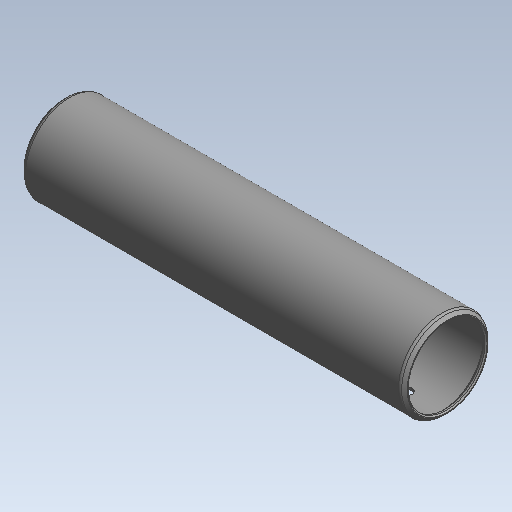
# Autodesk Inventor part: 04-3.4462C
Saved by Autodesk Inventor 2020 (Build 240168000, 168)
## iProperties
Part Number: 04-3.4462C
Material: Generic
Catalog Web Link: www.cadenas.de
Description: Tube-Original Line - Standard Air Cylinders
Vendor: BIMBA
Document SubType Name: Modeling
Designer: partserver
Manufacturer: BIMBA
Mass: 3.10241 g
Surface Area: 111.945 cm^2
Volume: 3.10241 cm^3
Density: 1 g/cm^3
Appearance: PSOLRGB-180-180-180
Category: PARTsolutions
Company: BIMBA
PSOL_IDENT_0: {$CADENAS_DATA\23d-libs\bimba\bimba_brand\bimba_imperial\bimba_full_line\original_line_cylinders\sta
PSOL_IDENT_1: ndard_air_cylinders\tube.prj},199 {VTYP=3D},{NB=04-3.4462C},{LINA=04-3.4462C},{NN=Tube},{DATE=19.01.
PSOL_IDENT_2: 2022 10:19:38},{GEOMDATE=03.03.2020 12:52:40},{VERSION=},{LINEID=40},{WBVAR=MNT,ACTING,NR,L,FOURHOLE
PSOL_IDENT_3: S,SR,K},{WBNUMERIC=L,FOURHOLES}  {NB=04-3.4462C},{LINA=04-3.4462C},{KT=DUMMY},{PN=04-3.4462C},{BORE=
PSOL_IDENT_4: 0.75000000},{BOREPN=04},{MNT=},{MNTALG='' , 'Front Nose' , 'BF' , 'Front Block' , 'BFT' , 'Front Tru
PSOL_IDENT_5: nnion' , 'A' , 'Adjustable Stroke'},{ACTING=},{ACTINGALG= '' , 'Single Acting' , 'R' , 'Reverse/Doub
PSOL_IDENT_6: le Acting' },{NR=},{NRALG= '' , 'Without Non-rotating Rod' , 'NR' , 'With Non-rotating Rod' },{L=3.4
PSOL_IDENT_7: 460},{OD=0.8050},{ODN=0.8050},{ODP=0.8625},{ODB=0.8325},{ID=0.7615},{DV=0.00000000},{LV=0.00000000},
PSOL_IDENT_8: {LV1=0.00000000},{G=0.0300},{FOURHOLES=2},{AA=0.3750},{BB=0.0940},{SR=C},{SRALG= 'C' , 'Carbon Steel
PSOL_IDENT_9: Rod' , 'SR' , '303 Stainless Steel Rod' , '' , '303 Stainless Steel Rod'},{KALG= '', 'Standard' , '
PSOL_IDENT_10: K' , 'Ports Rotated 90deg' },{K=}
NB: 04-3.4462C
NN: Tube
NT: Original Line - Standard Air Cylinders
NBSYN: $PN.
LINA: 04-3.4462C
CATALOG: Bimba Products
BORE: 0
BOREPN: 04
MNT: Front Nose
MNTALG: '' , 'Front Nose' , 'BF' , 'Front Block' , 'BFT' , 'Front Trunnion' , 'A' , 'Adjustable Stroke'
ACTING: Single Acting
NR: Without Non-rotating Rod
L: 3.446
ODN: 0.805
ODP: 0.8625
ODB: 0.8325
ID: 0.7615
DV: 0
LV: 0
LV1: 0
G: 0.03
FOURHOLES: 2
AA: 0.375
BB: 0.094
SR: Carbon Steel Rod
K: Standard
SUPPLIER: BIMBA
ARTICLENO: 04-3.4462C
BOMINFO: 04-3.4462C
CREATOR: CADENAS GmbH
Title: 04-3.4462C
Author: Cadenas PARTsolutions
Comments: Original Line - Standard Air Cylinders
Autodesk Inventor part; units mm, degrees
sketch "Sketch_1" plane through (0, 0, 0) normal (0, 0, 1) x (1, 0, 0)
  line L0 (87.5284, 0) -> (0, 0)
  arc A0 (-0.6395, 9.3472) -> (-0.6395, 9.1676) centre (-0.5497, 9.2574) ccw
  line L1 (-0.6395, 9.1676) -> (-0.381, 8.9091)
  line L2 (-0.381, 8.9091) -> (0, 8.9091)
  line L3 (0, 8.9091) -> (0.762, 9.671)
  line L4 (0.762, 9.671) -> (86.7664, 9.671)
  line L5 (86.7664, 9.671) -> (87.5284, 8.9091)
  line L6 (87.5284, 8.9091) -> (87.9094, 8.9091)
  line L7 (87.9094, 8.9091) -> (88.1679, 9.1676)
  arc A1 (88.1679, 9.1676) -> (88.1679, 9.3472) centre (88.0781, 9.2574) ccw
  line L8 (88.1679, 9.3472) -> (87.5148, 10.0003)
  arc A2 (87.5148, 10.0003) -> (86.9759, 10.2235) centre (86.976, 9.4615) ccw
  line L9 (86.9759, 10.2235) -> (0.5524, 10.2235)
  arc A3 (0.5524, 10.2235) -> (0.0136, 10.0003) centre (0.5524, 9.4615) ccw
  line L10 (0.0136, 10.0003) -> (-0.6395, 9.3472)
  constraints: 22 end point, 8 point on circle, 4 centre point
revolve "Revolution1" add sketch "Sketch_1" angle 360 about axis through (87.5284, 0, 0) along (1, 0, 0)
sketch "Sketch_4" plane through (0, 0, 0) normal (0, 0, 1) x (1, 0, 0)
  circle A0 centre (8.763, 0) radius 1.1938
  constraints: 1 centre point
extrude "Extrusion1" cut sketch "Sketch_4" along normal blind 10.2235
ref_plane "cp1_XY" through (43.7642, 0, 10.2235) normal (1, 0, 0) x (0, 0, -1)
ref_plane "cp1_YZ" through (43.7642, 0, 10.2235) normal (0, 0, -1) x (0, 1, 0)
ref_plane "cp1_ZX" through (43.7642, 0, 10.2235) normal (0, 1, 0) x (1, 0, 0)
ref_plane "cp2_XY" through (43.7642, 10.2235, 0) normal (1, 0, 0) x (0, 0, -1)
ref_plane "cp2_YZ" through (43.7642, 10.2235, 0) normal (0, 0, -1) x (0, 1, 0)
ref_plane "cp2_ZX" through (43.7642, 10.2235, 0) normal (0, 1, 0) x (1, 0, 0)
ref_plane "cp3_XY" through (43.7642, 0, -10.2235) normal (1, 0, 0) x (0, 0, -1)
ref_plane "cp3_YZ" through (43.7642, 0, -10.2235) normal (0, 0, -1) x (0, 1, 0)
ref_plane "cp3_ZX" through (43.7642, 0, -10.2235) normal (0, 1, 0) x (1, 0, 0)
ref_plane "cp4_XY" through (43.7642, -10.2235, 0) normal (1, 0, 0) x (0, 0, -1)
ref_plane "cp4_YZ" through (43.7642, -10.2235, 0) normal (0, 0, -1) x (0, 1, 0)
ref_plane "cp4_ZX" through (43.7642, -10.2235, 0) normal (0, 1, 0) x (1, 0, 0)
ref_plane "tube_front_XY" through (0, 0, 0) normal (1, 0, 0) x (0, 0, -1)
ref_plane "tube_front_YZ" through (0, 0, 0) normal (0, 0, -1) x (0, 1, 0)
ref_plane "tube_front_ZX" through (0, 0, 0) normal (0, 1, 0) x (1, 0, 0)
ref_plane "tube_rear_XY" through (87.5284, 0, 0) normal (1, 0, 0) x (0, 0, -1)
ref_plane "tube_rear_YZ" through (87.5284, 0, 0) normal (0, 0, -1) x (0, 1, 0)
ref_plane "tube_rear_ZX" through (87.5284, 0, 0) normal (0, 1, 0) x (1, 0, 0)
body "Solid1"
